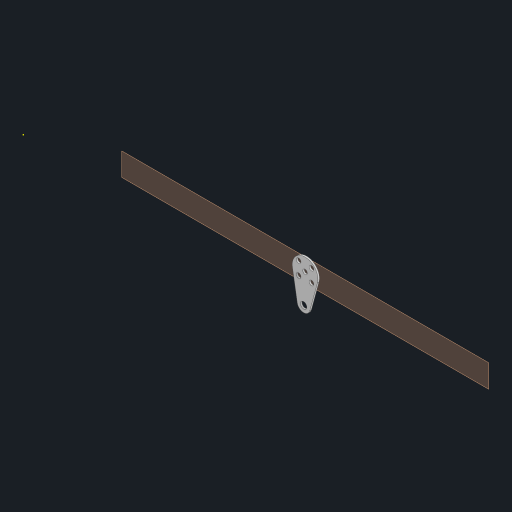
# Autodesk Inventor part: raised gear
Saved by Autodesk Inventor 2023 (Build 270158000, 158)
## iProperties
Created: 2023-06-19
Part Number: raised gear
Material: Generic
Document SubType Name: Modeling
Designer: reima
Density: 1 g/cm^3
Appearance: Default
Author: reima
Autodesk Inventor part; units mm, degrees
ref_plane "YZ Plane" through (0, 0, 0) normal (1, 0, 0) x (0, 1, 0)
ref_plane "XZ Plane" through (0, 0, 0) normal (0, 1, 0) x (-1, 0, 0)
ref_plane "XY Plane" through (0, 0, 0) normal (0, 0, 1) x (1, 0, 0)
ref_plane "Work Plane1" through (-1.4224, 0, 0) normal (0, 0, 1) x (1, 0, 0)
sketch "Sketch1" plane through (-1.4224, 0, 0) normal (0, 0, 1) x (1, 0, 0)
  circle A0 centre (280.3224, 21.9203) radius 2.3114 projected
  circle A1 centre (273.9724, 28.2703) radius 2.3114 projected
  circle A2 centre (286.6724, 28.2703) radius 2.3114 projected
  circle A3 centre (278.9, -7.4485) radius 2.3114 projected
  circle A4 centre (273.9724, 15.5703) radius 2.3114 projected
  circle A5 centre (286.6724, 15.5703) radius 2.3114 projected
  arc A6 (292.5755, 18.5809) -> (267.804, 19.7807) centre (280.3224, 21.9203) ccw
  arc A7 (272.6408, -8.5183) -> (285.0265, -9.1182) centre (278.9, -7.4485) ccw
  line L0 (285.0265, -9.1182) -> (292.5755, 18.5809)
  line L1 (272.6408, -8.5183) -> (267.804, 19.7807)
  circle A8 centre (280.3224, 21.9203) radius 2.3114
  circle A9 centre (273.9724, 15.5703) radius 2.3114
  circle A10 centre (286.6724, 15.5703) radius 2.3114
  point P0 (1.4224, 0)
  dimension "d0" = 25.4
  dimension "d1" = 12.7
  constraints: 5 centre point, 5 coincident, 4 end point, 4 point on circle, 4 tangent, 3 concentric
  measures "d0" diameter of A6
  measures "d1" diameter of A7
extrude "Extrusion1" add sketch "Sketch1" along normal blind 1.5875 contours A0 | L0 A7 L1 A6
sketch "Sketch2" plane through (-1.4224, 0, 1.5875) normal (0, 0, 1) x (1, 0, 0)
  point P0 (1.4224, 0)
sketch "Sketch3" plane through (-1.4224, 0, 1.5875) normal (0, 0, 1) x (1, 0, 0)
  circle A0 centre (278.9, -7.4485) radius 2.3114 projected
  circle A1 centre (278.9, -7.4485) radius 3.175
  point P0 (1.4224, 0)
  dimension "d4" = 6.35
  constraints: 1 centre point, 1 coincident
  measures "d4" diameter of A1
sketch "Sketch4" plane through (-1.4224, 0, 1.5875) normal (0, 0, 1) x (1, 0, 0)
  point P0 (1.4224, 0)
sketch "Sketch5" plane through (-1.4224, 0, 1.5875) normal (0, 0, 1) x (1, 0, 0)
  circle A0 centre (273.9724, 28.2703) radius 2.3114 projected
  circle A1 centre (273.9724, 28.2703) radius 2.3114
  circle A2 centre (286.6724, 28.2703) radius 2.3114 projected
  circle A3 centre (286.6724, 15.5703) radius 2.3114 projected
  circle A4 centre (273.9724, 15.5703) radius 2.3114 projected
  line L0 (273.9724, 28.2703) -> (286.6724, 15.5703)
  line L1 (286.6724, 15.5703) -> (286.6724, 28.2703)
  line L2 (286.6724, 28.2703) -> (273.9724, 15.5703)
  circle A5 centre (280.3224, 21.9203) radius 2.2479
  point P0 (1.4224, 0)
  dimension "d5" = 4.4958
  constraints: 6 end point, 2 centre point, 1 coincident, 1 midpoint, 1 perpendicular, 1 vertical
  measures "d5" diameter of A5
extrude "Extrusion2" cut sketch "Sketch3" against normal blind 1.5875 contours A0 | A1
extrude "Extrusion3" cut sketch "Sketch5" against normal blind 1.5875 contours A5 L2 L0 | L0 L2 A5 | L2 A5 L0 | L0 A5 L2
body "Solid1"
